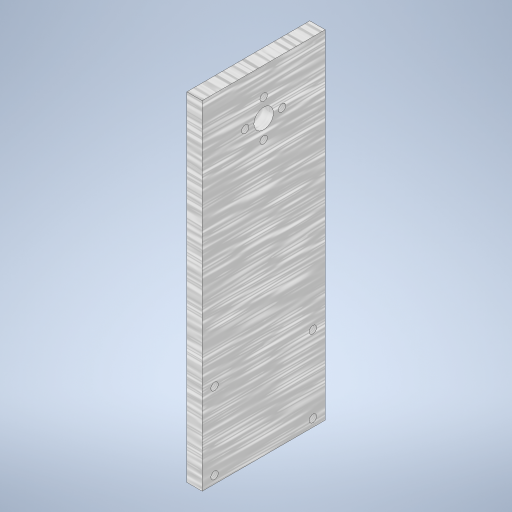
# Autodesk Inventor part: shoulder1_upper_cover
Saved by Autodesk Inventor 2024 (Build 280153000, 153)
## iProperties
Created: 2025-08-06
Part Number: shoulder1_upper_cover
Material: アルミニウム 5052
Document SubType Name: Modeling
Designer: HosodaLab2
Density: 2.68 g/cm^3
Appearance: サテン - ブラシ仕上げ 重厚
個数: 1
Author: HosodaLab2
Autodesk Inventor part; units mm, degrees
ref_plane "YZ Plane" through (0, 0, 0) normal (1, 0, 0) x (0, 1, 0)
ref_plane "XZ Plane" through (0, 0, 0) normal (0, 1, 0) x (-1, 0, 0)
ref_plane "XY Plane" through (0, 0, 0) normal (0, 0, 1) x (1, 0, 0)
sketch "スケッチ1" plane through (0, 0, 0) normal (0, 1, 0) x (-1, 0, 0)
  line L0 (0, 0) -> (-40, 0)
  line L1 (-40, 0) -> (-40, -110)
  line L2 (-40, -110) -> (0, -110)
  line L3 (0, -110) -> (0, 0)
  dimension "d0" = 40
  dimension "d1" = 110
  constraints: 8 end point, 2 parallel, 1 horizontal, 1 perpendicular
  measures "d0" distance of L2.end L1.end
  measures "d1" distance of L1.end L0.end
extrude "押し出し1" add sketch "スケッチ1" along normal blind 5
sketch "スケッチ2" plane through (0, 5, 0) normal (0, 1, 0) x (1, 0, 0)
  line L0 (0, 0) -> (40, 0) construction
  line L1 (20, 0) -> (20, 110) construction
  line L2 (40, 110) -> (0, 110) construction
  point P0 (20, 15)
  dimension "d4" = 15
  constraints: 2 end point, 2 midpoint, 1 point on line
  measures "d4" distance from line of L0 point (20, 15)
hole "穴1" at (20, 5, -15) direction (0, -1, 0) diameter 6.4 end through all
sketch "スケッチ3" plane through (0, 5, 0) normal (0, 1, 0) x (1, 0, 0)
  circle A0 centre (20, 15) radius 3.2 construction
  circle A1 centre (20, 15) radius 6 construction
  point P0 (0, 0)
  point P1 (14, 15)
  point P2 (20, 9)
  point P3 (26, 15)
  point P4 (20, 21)
  dimension "d12" = 12
  dimension "d15" = 360
  constraints: 1 coincident, 1 horizontal alignment, 7 other
hole "穴2" at (14, 5, -15) at (20, 5, -9) at (26, 5, -15) at (20, 5, -21) direction (0, -1, 0) diameter 2.459 end through all thread size "M3x0.5" class "6H" standard "ISO Metric profile"
sketch "スケッチ4" plane through (0, 5, 0) normal (0, 1, 0) x (1, 0, 0)
  line L0 (40, 110) -> (0, 110) construction
  line L1 (0, 110) -> (40, 110) construction
  line L2 (40, 110) -> (40, 105) construction
  line L3 (40, 105) -> (0, 105) construction
  line L4 (0, 105) -> (0, 110) construction
  line L5 (0, 110) -> (0, 0) projected
  line L6 (0, 107.5) -> (40, 107.5) construction
  line L7 (40, 0) -> (40, 110) projected
  line L8 (0, 110) -> (0, 0) construction
  line L9 (40, 80) -> (0, 80) construction
  line L10 (0, 80) -> (0, 85) construction
  line L11 (0, 85) -> (40, 85) construction
  line L12 (40, 85) -> (40, 80) construction
  line L13 (40, 82.5) -> (0, 82.5) construction
  point P0 (4, 107.5)
  point P1 (36, 107.5)
  point P2 (36, 82.5)
  point P3 (4, 82.5)
  dimension "d25" = 5
  dimension "d26" = 4
  dimension "d27" = 4
  dimension "d35" = 5
  dimension "d36" = 25
  constraints: 20 end point, 7 point on line, 4 parallel, 3 midpoint, 2 horizontal, 2 perpendicular
  measures "d25" distance of L1.end L2.end
  measures "d26" distance from line of point (4, 107.5) L5
  measures "d27" distance from line of L7 point (36, 107.5)
  measures "d35" distance of L9.end L10.end
  measures "d36" distance between parallel lines of L0 L11
hole "穴3" at (4, 5, -107.5) at (36, 5, -107.5) at (36, 5, -82.5) at (4, 5, -82.5) direction (0, -1, 0) diameter 2.459 end through all thread size "M3x0.5" class "6H" standard "ISO Metric profile"
